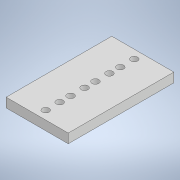
# Autodesk Inventor part: Assembly Plate
Saved by Autodesk Inventor 2022 (Build 260153000, 153)
## iProperties
Created: 2022-03-23
Part Number: Assembly Plate
Material: Generic
Document SubType Name: Modeling
Designer: Caleb
Density: 1 g/cm^3
Appearance: Default
Author: Caleb
Autodesk Inventor part; units mm, degrees
ref_plane "YZ Plane" through (0, 0, 0) normal (1, 0, 0) x (0, 1, 0)
ref_plane "XZ Plane" through (0, 0, 0) normal (0, 1, 0) x (-1, 0, 0)
ref_plane "XY Plane" through (0, 0, 0) normal (0, 0, 1) x (1, 0, 0)
sketch "Sketch1" plane through (0, 0, 0) normal (0, 1, 0) x (-1, 0, 0)
  line L0 (-63.5, -107.95) -> (63.5, -107.95)
  line L1 (63.5, -107.95) -> (63.5, 107.95)
  line L2 (63.5, 107.95) -> (-63.5, 107.95)
  line L3 (-63.5, 107.95) -> (-63.5, -107.95)
  line L4 (-63.5, -107.95) -> (63.5, 107.95) construction
  line L5 (63.5, -107.95) -> (-63.5, 107.95) construction
  point P0 (0, 0)
  dimension "d0" = 127
  dimension "d1" = 215.9
  constraints: 12 end point, 2 midpoint, 2 parallel, 1 horizontal, 1 perpendicular
  measures "d0" distance of L2.end L1.end
  measures "d1" distance of L1.end L0.end
extrude "Extrusion1" add sketch "Sketch1" along normal blind 19.05
sketch "Sketch4" plane through (0, 19.05, 0) normal (0, 1, 0) x (1, 0, 0)
  line L0 (-63.5, -107.95) -> (63.5, -107.95) projected
  line L1 (-63.5, 107.95) -> (-63.5, -107.95) projected
  point P0 (0, 0)
  point P1 (0, -90.5002)
  point P2 (0, -61.8871)
  point P3 (0, -11.0871)
  point P4 (0, -39.7002)
  point P5 (0, 39.7129)
  point P6 (0, 11.0998)
  point P7 (0, 90.5129)
  point P8 (0, 61.8998)
  dimension "d14" = 17.4498
  dimension "d15" = 46.0629
  dimension "d18" = 50.8
  constraints: 1 vertical, 6 other
  measures "d14" distance from line of L0 point (0, -90.5)
  measures "d15" distance from line of L0 point (0, -61.887)
  measures "d18" distance of point (0, -61.887) point (0, -11.087)
hole "Hole2" at (0, 19.05, 90.5002) at (0, 19.05, 61.8871) at (0, 19.05, 11.0871) at (0, 19.05, 39.7002) at (0, 19.05, -39.7129) at (0, 19.05, -11.0998) at (0, 19.05, -90.5129) at (0, 19.05, -61.8998) direction (0, -1, 0) diameter 3.9624 end through all counterbore diameter 13.97 counterbore depth 15.24 thread size "10-32 UNF" class "2B" standard "ANSI Unified Screw Threads"
body "Solid1"
